Autodesk Fusion 360 part; units mm, degrees
note: some values were not read from the file. Set by a fixed rule: which face or edge a step refers to.
(part 2 of 2)
sketch "Sketch34" plane through (453.263, -304.8, 0) normal (1, 0, 0) x (0, 1, 0)
  line L0 (0, 0) -> (-152.4, 0) construction
  line L1 (0, -18.288) -> (0, 0) construction
  line L2 (0, 0) -> (-2.2451, -2.2451) construction
  circle A0 centre (-2.2451, -2.2451) radius 3.175
  dimension "d298" = 3.175
  constraint coincident L0.start L1.end
  constraint coincident L0.start A0
  measures "d298" distance of L0.start L2.end
sweep "Sweep2''" cut kept parallel profiles "Sketch34" along 1 edges at (462.407, -304.8, 0) section 1 on bodies 4 bodies 4 in component "LeftSide"
ref_plane "WorkPlane21" through (254, -304.8, 0) normal (1, 0, 0) x (0, 1, 0)
sketch "Sketch35" plane through (254, -304.8, 0) normal (1, 0, 0) x (0, 1, 0)
  line L0 (0, 0) -> (-152.4, 0) construction
  line L1 (0, -18.288) -> (0, 0) construction
  line L2 (0, 0) -> (-2.2451, -2.2451) construction
  circle A0 centre (-2.2451, -2.2451) radius 3.175
  dimension "d306" = 3.175
  constraint coincident L0.start L1.end
  constraint coincident L0.start A0
  measures "d306" distance of L0.start L2.end
sweep "Sweep1'''" cut kept parallel profiles "Sketch35" along 1 edges at (263.144, -304.8, 0) section 1 on bodies 5 bodies 5 in component "Divider"
ref_plane "WorkPlane22" through (272.288, -152.4, 0) normal (-1, 0, 0) x (0, -1, 0)
sketch "Sketch36" plane through (272.288, -152.4, 0) normal (-1, 0, 0) x (0, -1, 0)
  line L0 (-152.4, 0) -> (0, 0) construction
  line L1 (0, -18.288) -> (0, 0) construction
  line L2 (0, 0) -> (-2.2451, -2.2451) construction
  circle A0 centre (-2.2451, -2.2451) radius 3.175
  dimension "d314" = 3.175
  constraint coincident L0.end L1.end
  constraint coincident L0.end A0
  measures "d314" distance of L0.end L2.end
sweep "Sweep2'''" cut kept parallel profiles "Sketch36" along 1 edges at (263.144, -152.4, 0) section 1 on bodies 5 bodies 5 in component "Divider"
ref_plane "WorkPlane23" through (254, -152.4, 304.8) normal (1, 0, 0) x (0, 1, 0)
sketch "Sketch37" plane through (254, -152.4, 304.8) normal (1, 0, 0) x (0, 1, 0)
  line L0 (152.4, 0) -> (0, 0) construction
  line L1 (0, 18.288) -> (0, 0) construction
  line L2 (0, 0) -> (2.2451, 2.2451) construction
  circle A0 centre (2.2451, 2.2451) radius 3.175
  dimension "d322" = 3.175
  constraint coincident L0.end L1.end
  constraint coincident L0.end A0
  measures "d322" distance of L0.end L2.end
sweep "Sweep3''" cut kept parallel profiles "Sketch37" along 1 edges at (263.144, -152.4, 304.8) section 1 on bodies 5 bodies 5 in component "Divider"
ref_plane "WorkPlane24" through (272.288, -304.8, 304.8) normal (-1, 0, 0) x (0, -1, 0)
sketch "Sketch38" plane through (272.288, -304.8, 304.8) normal (-1, 0, 0) x (0, -1, 0)
  line L0 (0, 0) -> (152.4, 0) construction
  line L1 (0, 18.288) -> (0, 0) construction
  line L2 (0, 0) -> (2.2451, 2.2451) construction
  circle A0 centre (2.2451, 2.2451) radius 3.175
  dimension "d330" = 3.175
  constraint coincident L0.start L1.end
  constraint coincident L0.start A0
  measures "d330" distance of L0.start L2.end
sweep "Sweep4''" cut kept parallel profiles "Sketch38" along 1 edges at (263.144, -304.8, 304.8) section 1 on bodies 5 bodies 5 in component "Divider"
ref_plane "WorkPlane25" through (453.263, -152.4, 323.088) normal (0, 0, -1) x (-1, 0, 0)
sketch "Sketch39" plane through (453.263, -152.4, 323.088) normal (0, 0, -1) x (-1, 0, 0)
  line L0 (0, 152.4) -> (0, 0) construction
  line L1 (0, 0) -> (-18.288, 0) construction
  line L2 (0, 0) -> (-2.2451, 2.2451) construction
  circle A0 centre (-2.2451, 2.2451) radius 3.175
  dimension "d338" = 3.175
  constraint coincident L0.end L1.start
  constraint coincident L0.end A0
  measures "d338" distance of L0.end L2.end
sweep "Sweep1''''" cut kept parallel profiles "Sketch39" along 1 edges at (453.263, -152.4, 313.944) section 1 on bodies 6 bodies 6 in component "Shelf"
ref_plane "WorkPlane26" through (453.263, -304.8, 304.8) normal (0, 0, 1) x (1, 0, 0)
sketch "Sketch40" plane through (453.263, -304.8, 304.8) normal (0, 0, 1) x (1, 0, 0)
  line L0 (0, 0) -> (0, -152.4) construction
  line L1 (18.288, 0) -> (0, 0) construction
  line L2 (0, 0) -> (2.2451, -2.2451) construction
  circle A0 centre (2.2451, -2.2451) radius 3.175
  dimension "d346" = 3.175
  constraint coincident L0.start L1.end
  constraint coincident L0.start A0
  measures "d346" distance of L0.start L2.end
sweep "Sweep2''''" cut kept parallel profiles "Sketch40" along 1 edges at (453.263, -304.8, 313.944) section 1 on bodies 6 bodies 6 in component "Shelf"
ref_plane "WorkPlane27" through (254, -152.4, 304.8) normal (0, 0, 1) x (1, 0, 0)
sketch "Sketch41" plane through (254, -152.4, 304.8) normal (0, 0, 1) x (1, 0, 0)
  line L0 (0, 0) -> (18.288, 0) construction
  line L1 (0, -152.4) -> (0, 0) construction
  line L2 (0, 0) -> (2.2451, -2.2451) construction
  circle A0 centre (2.2451, -2.2451) radius 3.175
  dimension "d354" = 3.175
  constraint coincident L0.start L1.end
  constraint coincident L0.start A0
  measures "d354" distance of L0.start L2.end
sweep "Sweep3'''" cut kept parallel profiles "Sketch41" along 1 edges at (254, -152.4, 313.944) section 1 on bodies 6 bodies 6 in component "Shelf"
ref_plane "WorkPlane28" through (254, -304.8, 304.8) normal (0, 0, 1) x (1, 0, 0)
sketch "Sketch42" plane through (254, -304.8, 304.8) normal (0, 0, 1) x (1, 0, 0)
  line L0 (0, 0) -> (0, 147.9099) construction
  line L1 (18.288, 0) -> (0, 0) construction
  line L2 (0, 0) -> (2.2451, 2.2451) construction
  circle A0 centre (2.2451, 2.2451) radius 3.175
  dimension "d362" = 3.175
  constraint coincident L0.start L1.end
  constraint coincident L0.start A0
  measures "d362" distance of L0.start L2.end
sweep "Sweep4'''" cut kept parallel profiles "Sketch42" along 1 edges at (254, -304.8, 313.944) section 1 on bodies 6 bodies 6 in component "Shelf"
ref_plane "WorkPlane29" through (272.288, -304.8, 304.8) normal (0, 0, 1) x (1, 0, 0)
sketch "Sketch43" plane through (272.288, -304.8, 304.8) normal (0, 0, 1) x (1, 0, 0)
  line L0 (0, 0) -> (-13.7979, 0) construction
  line L1 (0, 152.4) -> (0, 0) construction
  line L2 (0, 0) -> (-2.2451, 2.2451) construction
  circle A0 centre (-2.2451, 2.2451) radius 3.175
  dimension "d370" = 3.175
  constraint coincident L0.start L1.end
  constraint coincident L0.start A0
  measures "d370" distance of L0.start L2.end
sweep "Sweep5''" cut kept parallel profiles "Sketch43" along 1 edges at (272.288, -304.8, 313.944) section 1 on bodies 6 bodies 6 in component "Shelf"
ref_plane "WorkPlane30" through (272.288, -152.4, 304.8) normal (0, 0, 1) x (1, 0, 0)
sketch "Sketch44" plane through (272.288, -152.4, 304.8) normal (0, 0, 1) x (1, 0, 0)
  line L0 (0, 0) -> (-13.7979, 0) construction
  line L1 (0, -147.9099) -> (0, 0) construction
  line L2 (0, 0) -> (-2.2451, -2.2451) construction
  circle A0 centre (-2.2451, -2.2451) radius 3.175
  dimension "d378" = 3.175
  constraint coincident L0.start L1.end
  constraint coincident L0.start A0
  measures "d378" distance of L0.start L2.end
sweep "Sweep6''" cut kept parallel profiles "Sketch44" along 1 edges at (272.288, -152.4, 313.944) section 1 on bodies 6 bodies 6 in component "Shelf"
ref_plane "WorkPlane31" through (0, -304.8, 323.088) normal (0, 0, -1) x (-1, 0, 0)
sketch "Sketch45" plane through (0, -304.8, 323.088) normal (0, 0, -1) x (-1, 0, 0)
  line L0 (0, 0) -> (0, -152.4) construction
  line L1 (18.288, 0) -> (0, 0) construction
  line L2 (0, 0) -> (2.2451, -2.2451) construction
  circle A0 centre (2.2451, -2.2451) radius 3.175
  dimension "d386" = 3.175
  constraint coincident L0.start L1.end
  constraint coincident L0.start A0
  measures "d386" distance of L0.start L2.end
sweep "Sweep7''" cut kept parallel profiles "Sketch45" along 1 edges at (0, -304.8, 313.944) section 1 on bodies 6 bodies 6 in component "Shelf"
ref_plane "WorkPlane32" through (0, -152.4, 304.8) normal (0, 0, 1) x (1, 0, 0)
sketch "Sketch46" plane through (0, -152.4, 304.8) normal (0, 0, 1) x (1, 0, 0)
  line L0 (0, 152.4) -> (0, 0) construction
  line L1 (-18.288, 0) -> (0, 0) construction
  line L2 (0, 0) -> (-2.2451, 2.2451) construction
  circle A0 centre (-2.2451, 2.2451) radius 3.175
  dimension "d394" = 3.175
  constraint coincident L0.end L1.end
  constraint coincident L0.end A0
  measures "d394" distance of L0.end L2.end
sweep "Sweep8''" cut kept parallel profiles "Sketch46" along 1 edges at (0, -152.4, 313.944) section 1 on bodies 6 bodies 6 in component "Shelf"
ref_plane "WorkPlane33" through (0, -304.8, 1382.776) normal (0, 0, -1) x (-1, 0, 0)
sketch "Sketch47" plane through (0, -304.8, 1382.776) normal (0, 0, -1) x (-1, 0, 0)
  line L0 (0, 0) -> (0, 152.4) construction
  line L1 (18.288, 0) -> (0, 0) construction
  line L2 (0, 0) -> (2.2451, 2.2451) construction
  circle A0 centre (2.2451, 2.2451) radius 3.175
  dimension "d402" = 3.175
  constraint coincident L0.start L1.end
  constraint coincident L0.start A0
  measures "d402" distance of L0.start L2.end
sweep "Sweep1'''''" cut kept parallel profiles "Sketch47" along 1 edges at (0, -304.8, 1373.632) section 1 on bodies 7 bodies 7 in component "Bottom"
ref_plane "WorkPlane34" through (0, -152.4, 1382.776) normal (0, 0, -1) x (-1, 0, 0)
sketch "Sketch48" plane through (0, -152.4, 1382.776) normal (0, 0, -1) x (-1, 0, 0)
  line L0 (0, 0) -> (18.288, 0) construction
  line L1 (0, -147.9099) -> (0, 0) construction
  line L2 (0, 0) -> (2.2451, -2.2451) construction
  circle A0 centre (2.2451, -2.2451) radius 3.175
  dimension "d410" = 3.175
  constraint coincident L0.start L1.end
  constraint coincident L0.start A0
  measures "d410" distance of L0.start L2.end
sweep "Sweep2'''''" cut kept parallel profiles "Sketch48" along 1 edges at (0, -152.4, 1373.632) section 1 on bodies 7 bodies 7 in component "Bottom"
ref_plane "WorkPlane35" through (288.163, -18.288, 1364.488) normal (0, 0, 1) x (1, 0, 0)
sketch "Sketch49" plane through (288.163, -18.288, 1364.488) normal (0, 0, 1) x (1, 0, 0)
  line L0 (0, 0) -> (0, 18.288) construction
  line L1 (-123.063, 0) -> (0, 0) construction
  line L2 (0, 0) -> (-2.2451, 2.2451) construction
  circle A0 centre (-2.2451, 2.2451) radius 3.175
  dimension "d418" = 3.175
  constraint coincident L0.start L1.end
  constraint coincident L0.start A0
  measures "d418" distance of L0.start L2.end
sweep "Sweep3''''" cut kept parallel profiles "Sketch49" along 1 edges at (288.163, -18.288, 1373.632) section 1 on bodies 7 bodies 7 in component "Bottom"
ref_plane "WorkPlane36" through (165.1, -18.288, 1382.776) normal (0, 0, -1) x (-1, 0, 0)
sketch "Sketch50" plane through (165.1, -18.288, 1382.776) normal (0, 0, -1) x (-1, 0, 0)
  line L0 (0, 0) -> (0, 18.288) construction
  line L1 (-118.5729, 0) -> (0, 0) construction
  line L2 (0, 0) -> (-2.2451, 2.2451) construction
  circle A0 centre (-2.2451, 2.2451) radius 3.175
  dimension "d426" = 3.175
  constraint coincident L0.start L1.end
  constraint coincident L0.start A0
  measures "d426" distance of L0.start L2.end
sweep "Sweep4''''" cut kept parallel profiles "Sketch50" along 1 edges at (165.1, -18.288, 1373.632) section 1 on bodies 7 bodies 7 in component "Bottom"
ref_plane "WorkPlane37" through (453.263, -304.8, 1382.776) normal (0, 0, -1) x (-1, 0, 0)
sketch "Sketch51" plane through (453.263, -304.8, 1382.776) normal (0, 0, -1) x (-1, 0, 0)
  line L0 (0, 0) -> (-18.288, 0) construction
  line L1 (0, 152.4) -> (0, 0) construction
  line L2 (0, 0) -> (-2.2451, 2.2451) construction
  circle A0 centre (-2.2451, 2.2451) radius 3.175
  dimension "d434" = 3.175
  constraint coincident L0.start L1.end
  constraint coincident L0.start A0
  measures "d434" distance of L0.start L2.end
sweep "Sweep5'''" cut kept parallel profiles "Sketch51" along 1 edges at (453.263, -304.8, 1373.632) section 1 on bodies 7 bodies 7 in component "Bottom"
ref_plane "WorkPlane38" through (453.263, -152.4, 1382.776) normal (0, 0, -1) x (-1, 0, 0)
sketch "Sketch52" plane through (453.263, -152.4, 1382.776) normal (0, 0, -1) x (-1, 0, 0)
  line L0 (0, 0) -> (0, -147.9099) construction
  line L1 (-18.288, 0) -> (0, 0) construction
  line L2 (0, 0) -> (-2.2451, -2.2451) construction
  circle A0 centre (-2.2451, -2.2451) radius 3.175
  dimension "d442" = 3.175
  constraint coincident L0.start L1.end
  constraint coincident L0.start A0
  measures "d442" distance of L0.start L2.end
sweep "Sweep6'''" cut kept parallel profiles "Sketch52" along 1 edges at (453.263, -152.4, 1373.632) section 1 on bodies 7 bodies 7 in component "Bottom"
ref_plane "WorkPlane39" through (0, 0, 1262.888) normal (0, -1, 0) x (1, 0, 0)
sketch "Sketch53" plane through (0, 0, 1262.888) normal (0, -1, 0) x (1, 0, 0)
  line L0 (-18.288, 0) -> (0, 0) construction
  line L1 (0, 0) -> (0, -50.8) construction
  line L2 (0, 0) -> (-2.2451, -2.2451) construction
  circle A0 centre (-2.2451, -2.2451) radius 3.175
  dimension "d450" = 3.175
  constraint coincident L0.end L1.start
  constraint coincident L0.end A0
  measures "d450" distance of L0.end L2.end
sweep "Sweep1''''''" cut kept parallel profiles "Sketch53" along 1 edges at (0, -9.144, 1262.888) section 1 on bodies 9 bodies 9 in component "BackSupport"
ref_plane "WorkPlane40" through (0, 0, 1313.688) normal (0, -1, 0) x (1, 0, 0)
sketch "Sketch54" plane through (0, 0, 1313.688) normal (0, -1, 0) x (1, 0, 0)
  line L0 (0, 50.8) -> (0, 0) construction
  line L1 (0, 0) -> (-18.288, 0) construction
  line L2 (0, 0) -> (-2.2451, 2.2451) construction
  circle A0 centre (-2.2451, 2.2451) radius 3.175
  dimension "d458" = 3.175
  constraint coincident L0.end L1.start
  constraint coincident L0.end A0
  measures "d458" distance of L0.end L2.end
sweep "Sweep2''''''" cut kept parallel profiles "Sketch54" along 1 edges at (0, -9.144, 1313.688) section 1 on bodies 9 bodies 9 in component "BackSupport"
ref_plane "WorkPlane41" through (165.1, 0, 1364.488) normal (0, -1, 0) x (1, 0, 0)
sketch "Sketch55" plane through (165.1, 0, 1364.488) normal (0, -1, 0) x (1, 0, 0)
  line L0 (-165.1, 0) -> (0, 0) construction
  line L1 (0, 0) -> (0, 18.288) construction
  line L2 (0, 0) -> (-2.2451, 2.2451) construction
  circle A0 centre (-2.2451, 2.2451) radius 3.175
  dimension "d466" = 3.175
  constraint coincident L0.end L1.start
  constraint coincident L0.end A0
  measures "d466" distance of L0.end L2.end
sweep "Sweep3'''''" cut kept parallel profiles "Sketch55" along 1 edges at (165.1, -9.144, 1364.488) section 1 on bodies 9 bodies 9 in component "BackSupport"
ref_plane "WorkPlane42" through (288.163, 0, 1364.488) normal (0, -1, 0) x (1, 0, 0)
sketch "Sketch56" plane through (288.163, 0, 1364.488) normal (0, -1, 0) x (1, 0, 0)
  line L0 (165.1, 0) -> (0, 0) construction
  line L1 (0, 0) -> (0, 18.288) construction
  line L2 (0, 0) -> (2.2451, 2.2451) construction
  circle A0 centre (2.2451, 2.2451) radius 3.175
  dimension "d474" = 3.175
  constraint coincident L0.end L1.start
  constraint coincident L0.end A0
  measures "d474" distance of L0.end L2.end
sweep "Sweep4'''''" cut kept parallel profiles "Sketch56" along 1 edges at (288.163, -9.144, 1364.488) section 1 on bodies 9 bodies 9 in component "BackSupport"
ref_plane "WorkPlane43" through (453.263, 0, 1313.688) normal (0, -1, 0) x (1, 0, 0)
sketch "Sketch57" plane through (453.263, 0, 1313.688) normal (0, -1, 0) x (1, 0, 0)
  line L0 (0, 0) -> (18.288, 0) construction
  line L1 (0, 50.8) -> (0, 0) construction
  line L2 (0, 0) -> (2.2451, 2.2451) construction
  circle A0 centre (2.2451, 2.2451) radius 3.175
  dimension "d482" = 3.175
  constraint coincident L0.start L1.end
  constraint coincident L0.start A0
  measures "d482" distance of L0.start L2.end
sweep "Sweep5''''" cut kept parallel profiles "Sketch57" along 1 edges at (453.263, -9.144, 1313.688) section 1 on bodies 9 bodies 9 in component "BackSupport"
ref_plane "WorkPlane44" through (453.263, 0, 1262.888) normal (0, -1, 0) x (1, 0, 0)
sketch "Sketch58" plane through (453.263, 0, 1262.888) normal (0, -1, 0) x (1, 0, 0)
  line L0 (0, 0) -> (0, -50.8) construction
  line L1 (18.288, 0) -> (0, 0) construction
  line L2 (0, 0) -> (2.2451, -2.2451) construction
  circle A0 centre (2.2451, -2.2451) radius 3.175
  dimension "d490" = 3.175
  constraint coincident L0.start L1.end
  constraint coincident L0.start A0
  measures "d490" distance of L0.start L2.end
sweep "Sweep6''''" cut kept parallel profiles "Sketch58" along 1 edges at (453.263, -9.144, 1262.888) section 1 on bodies 9 bodies 9 in component "BackSupport"
sketch "Sketch59" plane through (272.288, 0, 0) normal (1, 0, 0) x (0, 0, -1)
  arc A0 (-304.8, -309.2901) -> (-309.2901, -304.8) centre (-307.0451, -307.0451) ccw
  line L0 (-304.8, -309.2901) -> (-304.8, -457.2)
  line L1 (-304.8, -457.2) -> (0, -457.2)
  line L2 (0, -457.2) -> (0, -309.2901)
  arc A1 (4.4901, -304.8) -> (0, -309.2901) centre (2.2451, -307.0451) ccw
  line L3 (4.4901, -304.8) -> (18.288, -304.8)
  line L4 (18.288, -304.8) -> (18.288, -152.4)
  line L5 (18.288, -152.4) -> (4.4901, -152.4)
  arc A2 (0, -147.9099) -> (4.4901, -152.4) centre (2.2451, -150.1549) ccw
  line L6 (0, -147.9099) -> (0, 0)
  line L7 (0, 0) -> (-304.8, 0)
  line L8 (-304.8, 0) -> (-304.8, -147.9099)
  arc A3 (-309.2901, -152.4) -> (-304.8, -147.9099) centre (-307.0451, -150.1549) ccw
  line L9 (-309.2901, -152.4) -> (-323.088, -152.4)
  line L10 (-323.088, -152.4) -> (-323.088, -304.8)
  line L11 (-323.088, -304.8) -> (-309.2901, -304.8)
ref_plane "WorkPlane45" through (453.263, -18.288, 1262.888) normal (1, 0, 0) x (0, 1, 0)
sketch "Sketch60" plane through (453.263, -18.288, 1262.888) normal (1, 0, 0) x (0, 1, 0)
  line L0 (0, 0) -> (18.288, 0) construction
  line L1 (0, 50.8) -> (0, 0) construction
  line L2 (0, 0) -> (2.2451, 2.2451) construction
  circle A0 centre (2.2451, 2.2451) radius 3.175
  dimension "d498" = 3.175
  constraint coincident L0.start L1.end
  constraint coincident L0.start A0
  measures "d498" distance of L0.start L2.end
sweep "Sweep3''''''" cut kept parallel profiles "Sketch60" along 1 edges at (462.407, -18.288, 1262.888) section 1 on bodies 4 bodies 4 in component "LeftSide"
ref_plane "WorkPlane46" through (471.551, -18.288, 1313.688) normal (-1, 0, 0) x (0, -1, 0)
sketch "Sketch61" plane through (471.551, -18.288, 1313.688) normal (-1, 0, 0) x (0, -1, 0)
  line L0 (0, 0) -> (-18.288, 0) construction
  line L1 (0, -46.3099) -> (0, 0) construction
  line L2 (0, 0) -> (-2.2451, -2.2451) construction
  circle A0 centre (-2.2451, -2.2451) radius 3.175
  dimension "d506" = 3.175
  constraint coincident L0.start L1.end
  constraint coincident L0.start A0
  measures "d506" distance of L0.start L2.end
sweep "Sweep4''''''" cut kept parallel profiles "Sketch61" along 1 edges at (462.407, -18.288, 1313.688) section 1 on bodies 4 bodies 4 in component "LeftSide"
ref_plane "WorkPlane47" through (471.551, -152.4, 304.8) normal (-1, 0, 0) x (0, -1, 0)
sketch "Sketch62" plane through (471.551, -152.4, 304.8) normal (-1, 0, 0) x (0, -1, 0)
  line L0 (0, 0) -> (0, 18.288) construction
  line L1 (152.4, 0) -> (0, 0) construction
  line L2 (0, 0) -> (2.2451, 2.2451) construction
  circle A0 centre (2.2451, 2.2451) radius 3.175
  dimension "d514" = 3.175
  constraint coincident L0.start L1.end
  constraint coincident L0.start A0
  measures "d514" distance of L0.start L2.end
sweep "Sweep5'''''" cut kept parallel profiles "Sketch62" along 1 edges at (462.407, -152.4, 304.8) section 1 on bodies 4 bodies 4 in component "LeftSide"
ref_plane "WorkPlane48" through (471.551, -152.4, 323.088) normal (-1, 0, 0) x (0, -1, 0)
sketch "Sketch63" plane through (471.551, -152.4, 323.088) normal (-1, 0, 0) x (0, -1, 0)
  line L0 (0, 0) -> (0, -13.7979) construction
  line L1 (152.4, 0) -> (0, 0) construction
  line L2 (0, 0) -> (2.2451, -2.2451) construction
  circle A0 centre (2.2451, -2.2451) radius 3.175
  dimension "d522" = 3.175
  constraint coincident L0.start L1.end
  constraint coincident L0.start A0
  measures "d522" distance of L0.start L2.end
sweep "Sweep6'''''" cut kept parallel profiles "Sketch63" along 1 edges at (462.407, -152.4, 323.088) section 1 on bodies 4 bodies 4 in component "LeftSide"
ref_plane "WorkPlane49" through (471.551, -304.8, 323.088) normal (-1, 0, 0) x (0, -1, 0)
sketch "Sketch64" plane through (471.551, -304.8, 323.088) normal (-1, 0, 0) x (0, -1, 0)
  line L0 (0, 0) -> (0, -18.288) construction
  line L1 (-147.9099, 0) -> (0, 0) construction
  line L2 (0, 0) -> (-2.2451, -2.2451) construction
  circle A0 centre (-2.2451, -2.2451) radius 3.175
  dimension "d530" = 3.175
  constraint coincident L0.start L1.end
  constraint coincident L0.start A0
  measures "d530" distance of L0.start L2.end
sweep "Sweep7'''" cut kept parallel profiles "Sketch64" along 1 edges at (462.407, -304.8, 323.088) section 1 on bodies 4 bodies 4 in component "LeftSide"
ref_plane "WorkPlane50" through (471.551, -304.8, 304.8) normal (-1, 0, 0) x (0, -1, 0)
sketch "Sketch65" plane through (471.551, -304.8, 304.8) normal (-1, 0, 0) x (0, -1, 0)
  line L0 (0, 0) -> (-147.9099, 0) construction
  line L1 (0, 13.7979) -> (0, 0) construction
  line L2 (0, 0) -> (-2.2451, 2.2451) construction
  circle A0 centre (-2.2451, 2.2451) radius 3.175
  dimension "d538" = 3.175
  constraint coincident L0.start L1.end
  constraint coincident L0.start A0
  measures "d538" distance of L0.start L2.end
sweep "Sweep8'''" cut kept parallel profiles "Sketch65" along 1 edges at (462.407, -304.8, 304.8) section 1 on bodies 4 bodies 4 in component "LeftSide"
component "RightSide" placed x (1, 0, 0) y (0, 1, 0) z (0, 0, 1) at (0, 0, 0)
component "LeftSide" placed x (1, 0, 0) y (0, 1, 0) z (0, 0, 1) at (0, 0, 0)
component "Divider" placed x (1, 0, 0) y (0, 1, 0) z (0, 0, 1) at (0, 0, 0)
component "Shelf" placed x (1, 0, 0) y (0, 1, 0) z (0, 0, 1) at (0, 0, 0)
component "Bottom" placed x (1, 0, 0) y (0, 1, 0) z (0, 0, 1) at (0, 0, 0)
component "Back" placed x (1, 0, 0) y (0, 1, 0) z (0, 0, 1) at (0, 0, 0)
component "BackSupport" placed x (1, 0, 0) y (0, 1, 0) z (0, 0, 1) at (0, 0, 0)
component "Top" placed x (1, 0, 0) y (0, 1, 0) z (0, 0, 1) at (0, 0, 0)
equation "ply = 0.72 in"
equation "d4 = ply"
equation "d8 = ply"
equation "d9 = 17.125 in + ply * 3"
equation "d10 = 53 in + ply"
equation "d11 = 53 in + ply"
equation "d12 = 17.125 in + ply * 3"
equation "d13 = ply"
equation "d14 = 17.125 in + ply"
equation "d15 = ply"
equation "d28 = ply"
equation "d30 = ply"
equation "d31 = ply"
equation "d33 = ply * 2"
equation "d34 = ( 0.72 * 2 ) * 1 in"
equation "d36 = ( 0.72 * 2 ) * 1 in"
equation "d42 = ply * 2"
equation "d44 = ply * 2"
equation "d46 = ply * 2"
equation "d51 = 7.125 in + ply / 2"
equation "d52 = ply"
equation "d57 = ply * 2"
equation "d58 = ply * 2"
equation "d59 = ply * 2"
equation "d62 = ply * 1.5 + 7.125 in"
equation "d63 = ply"
equation "d67 = ply * 2"
equation "d68 = 12 in + ply / 2"
equation "d69 = ply"
equation "d71 = ply * 2"
equation "d77 = ply * 2"
equation "d79 = ply * 2"
equation "d81 = 12 in + ply / 2"
equation "d82 = ply"
equation "d88 = ply * 2"
equation "d90 = ply * 2"
equation "d93 = 12 in + ply * 1.5"
equation "d95 = ply"
equation "d97 = ply * 2"
equation "d99 = ply * 2"
equation "d100 = ply * 2"
equation "d102 = ply * 2"
equation "d107 = ply * 2"
equation "d111 = ply * 2"
equation "d120 = -ply"
equation "d121 = -ply"
equation "d122 = -ply"
equation "d123 = -ply"
equation "d124 = -ply"
equation "d146 = 0.25 in / 2 + 0.00 in"
equation "d154 = 0.25 in / 2 + 0.00 in"
equation "d162 = 0.25 in / 2 + 0.00 in"
equation "d170 = 0.25 in / 2 + 0.00 in"
equation "d178 = 0.25 in / 2 + 0.00 in"
equation "d186 = 0.25 in / 2 + 0.00 in"
equation "d194 = 0.25 in / 2 + 0.00 in"
equation "d202 = 0.25 in / 2 + 0.00 in"
equation "d210 = 0.25 in / 2 + 0.00 in"
equation "d218 = 0.25 in / 2 + 0.00 in"
equation "d226 = 0.25 in / 2 + 0.00 in"
equation "d234 = 0.25 in / 2 + 0.00 in"
equation "d242 = 0.25 in / 2 + 0.00 in"
equation "d250 = 0.25 in / 2 + 0.00 in"
equation "d258 = 0.25 in / 2 + 0.00 in"
equation "d266 = 0.25 in / 2 + 0.00 in"
equation "d274 = 0.25 in / 2 + 0.00 in"
equation "d282 = 0.25 in / 2 + 0.00 in"
equation "d290 = 0.25 in / 2 + 0.00 in"
equation "d298 = 0.25 in / 2 + 0.00 in"
equation "d306 = 0.25 in / 2 + 0.00 in"
equation "d314 = 0.25 in / 2 + 0.00 in"
equation "d322 = 0.25 in / 2 + 0.00 in"
equation "d330 = 0.25 in / 2 + 0.00 in"
equation "d338 = 0.25 in / 2 + 0.00 in"
equation "d346 = 0.25 in / 2 + 0.00 in"
equation "d354 = 0.25 in / 2 + 0.00 in"
equation "d362 = 0.25 in / 2 + 0.00 in"
equation "d370 = 0.25 in / 2 + 0.00 in"
equation "d378 = 0.25 in / 2 + 0.00 in"
equation "d386 = 0.25 in / 2 + 0.00 in"
equation "d394 = 0.25 in / 2 + 0.00 in"
equation "d402 = 0.25 in / 2 + 0.00 in"
equation "d410 = 0.25 in / 2 + 0.00 in"
equation "d418 = 0.25 in / 2 + 0.00 in"
equation "d426 = 0.25 in / 2 + 0.00 in"
equation "d434 = 0.25 in / 2 + 0.00 in"
equation "d442 = 0.25 in / 2 + 0.00 in"
equation "d450 = 0.25 in / 2 + 0.00 in"
equation "d458 = 0.25 in / 2 + 0.00 in"
equation "d466 = 0.25 in / 2 + 0.00 in"
equation "d474 = 0.25 in / 2 + 0.00 in"
equation "d482 = 0.25 in / 2 + 0.00 in"
equation "d490 = 0.25 in / 2 + 0.00 in"
equation "d498 = 0.25 in / 2 + 0.00 in"
equation "d506 = 0.25 in / 2 + 0.00 in"
equation "d514 = 0.25 in / 2 + 0.00 in"
equation "d522 = 0.25 in / 2 + 0.00 in"
equation "d530 = 0.25 in / 2 + 0.00 in"
equation "d538 = 0.25 in / 2 + 0.00 in"
